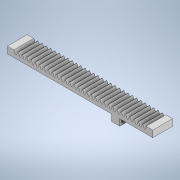
# Autodesk Inventor part: RACK
Saved by Autodesk Inventor 2021 (Build 250183000, 183)
## iProperties
Created: 2022-09-27
Part Number: RACK
Material: Generic
Document SubType Name: Modeling
Designer: ASUS
Density: 1 g/cm^3
Appearance: Default
Author: ASUS
Autodesk Inventor part; units mm, degrees
ref_plane "YZ Plane" through (0, 0, 0) normal (1, 0, 0) x (0, 1, 0)
ref_plane "XZ Plane" through (0, 0, 0) normal (0, 1, 0) x (-1, 0, 0)
ref_plane "XY Plane" through (0, 0, 0) normal (0, 0, 1) x (1, 0, 0)
sketch "Sketch1" plane through (0, 0, 0) normal (0, 0, 1) x (1, 0, 0)
  spline S0 degree 3 poles (-2.3918, 19.9824) (-2.3319, 19.9037) (-2.212, 19.7465) (-2.0415, 19.5038) (-1.8784, 19.2562) (-1.7238, 19.003) (-1.5786, 18.7444) (-1.4437, 18.4802) (-1.3205, 18.2104) (-1.2109, 17.9348) (-1.1332, 17.7) (-1.0819, 17.5091) (-1.0393, 17.3159) (-1.0179, 17.1189) (-0.97, 16.9268) (-0.9218, 16.7864) (-0.8588, 16.6519) (-0.7802, 16.5257) (-0.6986, 16.4324) (-0.6259, 16.3653) (-0.5659, 16.3216) (-0.5035, 16.2812) (-0.4363, 16.2497) (-0.3675, 16.2217) (-0.2954, 16.204) (-0.2225, 16.19) (-0.1235, 16.1859) (0, 16.1885) (0.1235, 16.1859) (0.2225, 16.19) (0.2954, 16.204) (0.3675, 16.2217) (0.4363, 16.2497) (0.5035, 16.2812) (0.5659, 16.3216) (0.6259, 16.3653) (0.6986, 16.4324) (0.7802, 16.5257) (0.8588, 16.6519) (0.9218, 16.7864) (0.97, 16.9268) (1.0179, 17.1189) (1.0393, 17.3159) (1.0819, 17.5091) (1.1332, 17.7) (1.2109, 17.9348) (1.3205, 18.2104) (1.4437, 18.4802) (1.5786, 18.7444) (1.7238, 19.003) (1.8784, 19.2562) (2.0415, 19.5038) (2.212, 19.7465) (2.3319, 19.9037) (2.3918, 19.9824) knots 0 0 0 0 0.029653 0.059306 0.088959 0.118612 0.148265 0.177917 0.207569 0.23722 0.266869 0.281695 0.29652 0.326167 0.340991 0.355815 0.370637 0.385456 0.400269 0.407684 0.415095 0.422509 0.429921 0.437334 0.444746 0.452159 0.45957 0.474397 0.489224 0.496635 0.504048 0.51146 0.518873 0.526285 0.533699 0.54111 0.548525 0.563338 0.578157 0.592978 0.607803 0.622627 0.652274 0.667099 0.681925 0.711574 0.741225 0.770877 0.800529 0.830182 0.859835 0.889488 0.919141 0.948794 0.948794 0.948794 0.948794
  circle A0 centre (0, 0) radius 16.1875 construction
  circle A1 centre (0, 0) radius 17.2669 construction
  circle A2 centre (0, 0) radius 18.375 construction
  line L0 (-2.3918, 19.9824) -> (2.3918, 19.9824)
  point P0 (-2.2136, 19.7454)
  point P1 (-2.0428, 19.503)
  point P2 (-1.8798, 19.2552)
  point P3 (-1.7254, 19.0021)
  point P4 (-1.5803, 18.7435)
  point P5 (-1.4456, 18.4793)
  point P6 (-1.3228, 18.2094)
  point P7 (-1.2136, 17.9337)
  point P8 (-1.1212, 17.652)
  point P9 (-1.083, 17.5088)
  point P10 (-1.0517, 17.3639)
  point P11 (-1.0037, 17.0713)
  point P12 (-0.968, 16.9274)
  point P13 (-0.9193, 16.7874)
  point P14 (-0.8562, 16.6533)
  point P15 (-0.777, 16.528)
  point P16 (-0.6798, 16.4163)
  point P17 (-0.6249, 16.3664)
  point P18 (-0.5655, 16.3221)
  point P19 (-0.5027, 16.2827)
  point P20 (-0.4361, 16.2503)
  point P21 (-0.367, 16.2234)
  point P22 (-0.2953, 16.2046)
  point P23 (-0.2223, 16.1918)
  point P24 (-0.1483, 16.1875)
  point P25 (0, 16.1875)
  point P26 (0.1483, 16.1875)
  point P27 (0.2223, 16.1918)
  point P28 (0.2953, 16.2046)
  point P29 (0.367, 16.2234)
  point P30 (0.4361, 16.2503)
  point P31 (0.5027, 16.2827)
  point P32 (0.5655, 16.3221)
  point P33 (0.6249, 16.3664)
  point P34 (0.6798, 16.4163)
  point P35 (0.777, 16.528)
  point P36 (0.8562, 16.6533)
  point P37 (0.9193, 16.7874)
  point P38 (0.968, 16.9274)
  point P39 (1.0037, 17.0713)
  point P40 (1.0517, 17.3639)
  point P41 (1.083, 17.5088)
  point P42 (1.1212, 17.652)
  point P43 (1.2136, 17.9337)
  point P44 (1.3228, 18.2094)
  point P45 (1.4456, 18.4793)
  point P46 (1.5803, 18.7435)
  point P47 (1.7254, 19.0021)
  point P48 (1.8798, 19.2552)
  point P49 (2.0428, 19.503)
  point P50 (2.2136, 19.7454)
  constraints: 3 centre point, 2 end point, 2 horizontal, 111 other
sketch "Sketch3" plane through (0, 0, 0) normal (0, 0, 1) x (1, 0, 0)
  line L0 (-10.3918, 19.9824) -> (157.6082, 19.9824)
  line L1 (157.6082, 19.9824) -> (157.6082, 11.9824)
  line L2 (157.6082, 11.9824) -> (-10.3918, 11.9824)
  line L3 (-10.3918, 11.9824) -> (-10.3918, 19.9824)
  point P0 (0, 0)
  point P1 (-2.3918, 19.9824)
  point P2 (2.3918, 19.9824)
  dimension "d16" = 168
  dimension "d17" = 8
  dimension "d18" = 8
  constraints: 8 end point, 2 parallel, 1 horizontal, 1 perpendicular, 1 point on line
  measures "d16" distance between parallel lines of L1 L3
  measures "d17" distance between parallel lines of L2 L0
  measures "d18" distance from line of L3 point (-2.392, 19.982)
extrude "Extrusion4" add sketch "Sketch3" against normal blind 24
extrude "Extrusion5" cut sketch "Sketch1" against normal through all
pattern_linear "Rectangular Pattern1" count 31 spacing 5.2 along (1, 0, 0) of "Extrusion5"
sketch "Sketch4" plane through (157.6082, 11.9824, 0) normal (1, 0, 0) x (0, 0, -1)
  line L0 (0, 8) -> (24, 8) projected
  line L1 (0, 0) -> (24, 0)
  line L2 (24, 0) -> (24, 8)
  line L3 (24, 8) -> (0, 8)
  line L4 (0, 8) -> (0, 0)
  point P0 (0, -11.9824)
  constraints: 8 end point, 2 parallel, 1 horizontal, 1 perpendicular
extrude "Extrusion6" add sketch "Sketch4" along normal blind 8
sketch "Sketch5" plane through (-10.3918, 11.9824, -24) normal (0, -1, 0) x (1, 0, 0)
  line L0 (136, 24) -> (126, 24)
  line L1 (126, 24) -> (126, 0)
  line L2 (126, 0) -> (136, 0)
  line L3 (136, 0) -> (136, 24)
  line L4 (176, 24) -> (176, 0) projected
  point P0 (10.3918, 24)
  dimension "d28" = 10
  dimension "d29" = 24
  dimension "d30" = 40
  constraints: 8 end point, 2 parallel, 1 horizontal, 1 perpendicular
  measures "d28" distance of L2.end L1.end
  measures "d29" distance between parallel lines of L2 L0
  measures "d30" distance between parallel lines of L4 L3
extrude "Extrusion7" add sketch "Sketch5" along normal blind 8
sketch "Sketch6" plane through (125.6082, 11.9824, 0) normal (1, 0, 0) x (0, 0, -1)
  circle A0 centre (20, -4) radius 2.05
  circle A1 centre (4, -4) radius 2.05
  line L0 (24, -8) -> (0, -8) projected
  line L1 (24, 0) -> (24, -8) projected
  line L2 (0, 0) -> (0, -8) projected
  point P0 (0, -11.9824)
  dimension "d33" = 4.1
  dimension "d34" = 4.1
  dimension "d35" = 4
  dimension "d36" = 4
  dimension "d37" = 4
  dimension "d38" = 4
  constraints: 2 centre point
  measures "d33" diameter of A0
  measures "d34" diameter of A1
  measures "d35" distance from line of L0 A0.centre
  measures "d36" distance from line of L1 A0.centre
  measures "d37" distance from line of L2 A1.centre
  measures "d38" distance from line of L0 A1.centre
extrude "Extrusion8" cut sketch "Sketch6" against normal through all
equation "\"Module\" = 1.75"
equation "\"PressureAngle\" = 20deg"
equation "\"UnitProfileClearance\" = 0.25"
equation "\"UnitRoundRadius\" = 0.35"
equation "\"HeadDiameter\" = 40.25"
equation "\"RootDiameter\" = 32.375"
equation "\"BaseDiameter\" = 34.5337"
equation "\"PitchDiameter\" = 36.75"
equation "\"FaceWidth\" = 24"
equation "\"HelixAngle\" = 0"
equation "\"UnitCorrection\" = 0"
equation "\"UnitAddendumModification\" = 0"
equation "\"CircularPitch\" = 5.497787"
equation "\"UnitBacklashShift\" = 0"
equation "\"TotalToolShift\" = 0"
equation "\"IsInternal\" = 0"
body "Solid2"
